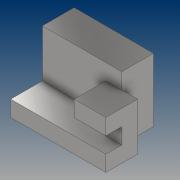
# Autodesk Inventor part: 11
Saved by Autodesk Inventor 2020.2 (Build 242310000, 310)
## iProperties
Created: 2020-09-17
Part Number: 11
Material: 鋼、碳鋼
Document SubType Name: Modeling
Designer: user
Density: 7.85 g/cm^3
Appearance: 半拋光
Mass: 455.3 g
Surface Area: 120 cm^2
Volume: 58 cm^3
Author: user
Autodesk Inventor part; units mm, degrees
ref_plane "YZ Plane" through (0, 0, 0) normal (1, 0, 0) x (0, 1, 0)
ref_plane "XZ Plane" through (0, 0, 0) normal (0, 1, 0) x (-1, 0, 0)
ref_plane "XY Plane" through (0, 0, 0) normal (0, 0, 1) x (1, 0, 0)
sketch "草圖1" plane through (0, 0, 0) normal (0, 1, 0) x (-1, 0, 0)
  line L0 (0, 0) -> (-60, 0)
  line L1 (-60, 0) -> (-60, -40)
  line L2 (-60, -40) -> (0, -40)
  line L3 (0, -40) -> (0, 0)
  dimension "d0" = 60
  dimension "d1" = 40
  constraints: 8 end point, 2 parallel, 1 horizontal, 1 perpendicular
  measures "d0" distance of L0.start L0.end
  measures "d1" distance of L2.end L0.start
extrude "擠出1" add sketch "草圖1" along normal blind 40
sketch "草圖2" plane through (60, 0, 0) normal (1, 0, 0) x (0, 0, -1)
  line L0 (40, 0) -> (40, 40) projected
  line L1 (40, 0) -> (20, 0)
  line L2 (20, 0) -> (20, 55.5046)
  line L3 (20, 55.5046) -> (40, 55.5046)
  line L4 (40, 55.5046) -> (40, 0)
  point P0 (0, 0)
  point P1 (40, 40)
  dimension "d4" = 20
  constraints: 8 end point, 2 parallel, 1 horizontal, 1 perpendicular
  measures "d4" distance of L2.end L3.end
extrude "擠出2" cut sketch "草圖2" against normal blind 10
sketch "草圖3" plane through (0, 0, 0) normal (0, 0, 1) x (1, 0, 0)
  line L0 (0, 40) -> (60, 40) projected
  line L1 (60, 40) -> (60, 0) projected
  line L2 (60, 0) -> (0, 0) projected
  line L3 (0, 0) -> (0, 40) projected
  line L4 (0, 0) -> (0, 40) projected
  line L5 (0, 10) -> (40, 10)
  line L6 (40, 10) -> (40, 30)
  line L7 (40, 30) -> (60, 30)
  line L8 (60, 0) -> (60, 40) projected
  dimension "d7" = 10
  dimension "d8" = 20
  dimension "d9" = 10
  constraints: 6 end point, 2 perpendicular, 2 point on line, 1 horizontal
  measures "d7" distance between parallel lines of L7 L0
  measures "d8" distance between parallel lines of L1 L6
  measures "d9" distance between parallel lines of L2 L5
extrude "擠出3" cut sketch "草圖3" against normal blind 20 contours L0 L1 L7 L6 L5 L3
sketch "草圖4" plane through (40, 10, 0) normal (-1, 0, 0) x (0, 0, 1)
  line L0 (-20, 30) -> (-20, 20) projected
  line L1 (-20, 20) -> (-20, 0) projected
  line L2 (-20, 0) -> (0, 0) projected
  line L3 (0, 20) -> (0, 0) projected
  line L4 (-20, 20) -> (0, 20) projected
  line L5 (-40, 30) -> (-20, 30) projected
  line L6 (-40, -10) -> (-40, 30) projected
  line L7 (0, -10) -> (-40, -10) projected
  line L8 (0, 0) -> (0, -10) projected
  line L9 (0, 20) -> (0, 0) projected
  line L10 (0, 10) -> (-10, 10)
  line L11 (-10, 10) -> (-10, 0)
  line L12 (-10, 0) -> (0, 0)
  line L13 (0, 0) -> (0, 10)
  point P0 (-10, 0)
  dimension "d12" = 10
  dimension "d13" = 10
  dimension "d14" = 10
  constraints: 8 end point, 2 parallel, 1 horizontal, 1 midpoint, 1 perpendicular
  measures "d12" distance of L10.start L10.end
  measures "d13" distance between parallel lines of L7 L12
  measures "d14" distance of L10.end L11.end
extrude "擠出4" cut sketch "草圖4" against normal blind 28 contours L11 L10 L3 L2
